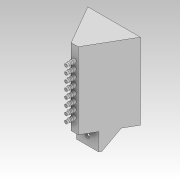
# Autodesk Inventor part: Manifold_8
Saved by Autodesk Inventor 2020 (Build 240168000, 168)
## iProperties
Created: 2020-08-02
Part Number: Manifold_8
Material: Generic
Document SubType Name: Modeling
Designer: DDeGo
Density: 1 g/cm^3
Appearance: Default
Author: DDeGo
Autodesk Inventor part; units mm, degrees
ref_plane "YZ Plane" through (0, 0, 0) normal (1, 0, 0) x (0, 1, 0)
ref_plane "XZ Plane" through (0, 0, 0) normal (0, 1, 0) x (-1, 0, 0)
ref_plane "XY Plane" through (0, 0, 0) normal (0, 0, 1) x (1, 0, 0)
sketch "Sketch1" plane through (0, 0, 0) normal (1, 0, 0) x (0, 1, 0)
  line L0 (1.75, 10) -> (1.05, 10)
  line L1 (0, 0) -> (0, 10) construction
  line L2 (0, 10) -> (1.05, 10) construction
  line L3 (1.8198, 8) -> (2.2759, 6.4097)
  line L4 (2.2759, 6.4097) -> (1.8759, 6.3957)
  line L5 (1.9282, 4.8957) -> (2.3843, 3.3053)
  line L6 (2.3843, 3.3053) -> (1.9843, 3.2914)
  line L7 (1.8759, 6.3957) -> (1.8198, 8) construction
  line L8 (1.8198, 8) -> (1.75, 10)
  line L9 (1.9282, 4.8957) -> (1.8759, 6.3957)
  line L10 (1.9843, 3.2914) -> (1.9282, 4.8957) construction
  line L11 (2.0992, 0) -> (1.9843, 3.2914)
  line L12 (1.05, 10) -> (1.05, 0)
  line L13 (1.05, 0) -> (2.0992, 0)
  line L14 (1.05, 0) -> (0, 0) construction
  dimension "d0" = 1.75
  dimension "d1" = 0.7
  dimension "d3" = 0.4
  dimension "d5" = 10
  dimension "d6" = 2
  dimension "d7" = 1.5
  dimension "d14" = 14
  dimension "d48" = 2
  constraints: 30 end point, 12 perpendicular, 2 horizontal, 2 parallel, 2 vertical
  measures "d0" distance of L1.end L0.start
  measures "d1" distance of L0.start L0.end
  measures "d3" horizontal distance of L3.end L4.end
  measures "d5" vertical distance of L11.start L0.start
  measures "d6" vertical distance of L0.end L3.start
  measures "d7" vertical distance of L4.end L5.start
  measures "d14" angle of L3 L7
  measures "d48" angle of L12 L8
revolve "Revolution1" add sketch "Sketch1" angle 360 about axis through (0, 0, 0) along (0, 0, 1)
pattern_linear "Rectangular Pattern1" count 8 spacing 8 along (0, 1, 0) of "Revolution1"
sketch "Sketch5" plane through (0, 0, 0) normal (0, 0, -1) x (-1, 0, 0)
  line L0 (4, 60) -> (-4, 60)
  line L1 (-4, 60) -> (-4, -4)
  line L2 (-4, -4) -> (4, -4)
  line L3 (4, -4) -> (4, 60)
  circle A0 centre (0, 56) radius 1.05 projected
  circle A1 centre (0, 48) radius 1.05 projected
  circle A2 centre (0, 40) radius 1.05 projected
  circle A3 centre (0, 32) radius 1.05 projected
  circle A4 centre (0, 24) radius 1.05 projected
  circle A5 centre (0, 16) radius 1.05 projected
  circle A6 centre (0, 8) radius 1.05 projected
  circle A7 centre (0, 0) radius 1.05 projected
  dimension "d50" = 4
  dimension "d51" = 4
  dimension "d55" = 4
  dimension "d56" = 4
  constraints: 8 end point, 2 parallel, 1 horizontal, 1 perpendicular
  measures "d50" distance from line of point (0, 0) L3
  measures "d51" distance from line of L1 point (0, 0)
  measures "d55" distance from line of L0 A0.centre
  measures "d56" distance from line of L2 point (0, 0)
extrude "Extrusion3" add sketch "Sketch5" along normal blind 8
ref_plane "Work Plane1" through (0, 0, -4) normal (0, 0, -1) x (-1, 0, 0)
sketch "Sketch6" plane through (-4, -4, 0) normal (0, -1, 0) x (1, 0, 0)
  line L0 (5.05, -8) -> (2.95, -8) construction
  circle A0 centre (4, -4) radius 1.75
  line L1 (9.6, -4) -> (-1.6, -4) construction
  line L2 (8, -8) -> (0, -8) projected
  line L3 (4, -8) -> (4, 0) construction
  dimension "d59" = 3.5
  constraints: 3 midpoint, 2 end point, 1 centre point, 1 coincident, 1 vertical
  measures "d59" diameter of A0
extrude "Extrusion4" cut sketch "Sketch6" against normal through all
sketch "Sketch7" plane through (0, 0, -8) normal (0, 0, -1) x (-1, 0, 0)
  circle A0 centre (0, 0) radius 1.05 projected
  line L0 (4, -4) -> (4, 60) projected
  line L1 (4, 60) -> (-4, 60) projected
  line L2 (-4, 60) -> (-4, -4) projected
  line L3 (-4, -4) -> (4, -4) projected
  circle A1 centre (0, 0) radius 1.05 projected
  circle A2 centre (0, 8) radius 1.05 projected
  circle A3 centre (0, 16) radius 1.05 projected
  circle A4 centre (0, 24) radius 1.05 projected
  circle A5 centre (0, 32) radius 1.05 projected
  circle A6 centre (0, 40) radius 1.05 projected
  circle A7 centre (0, 48) radius 1.05 projected
  circle A8 centre (0, 56) radius 1.05 projected
extrude "Extrusion5" add sketch "Sketch7" against normal up to surface contours A0 | A2 | A3 | A4 | A5 | A6 | A7 | A8 round surface about axis through (0, -4, -4) along (0, 1, 0) radius 1.75 far side no
sketch "Sketch10" plane through (-4, -4, 0) normal (0, -1, 0) x (1, 0, 0)
  line L0 (20.3187, -16.469) -> (-14.4175, -16.469)
  line L1 (-14.4175, -16.469) -> (-14.4175, -4)
  line L2 (-14.4175, -4) -> (20.3187, -4)
  line L3 (20.3187, -4) -> (20.3187, -16.469)
  circle A0 centre (4, -4) radius 1.75 projected
  point P0 (4, 0)
  constraints: 8 end point, 2 parallel, 1 horizontal, 1 perpendicular, 1 point on line
extrude "Extrusion6" cut sketch "Sketch10" against normal through all contours L0 L1 L2 A0 L3 | A0 L2 picked at (3.6188, -4.8908)
sketch "Sketch11" plane through (-4, -4, 0) normal (0, -1, 0) x (1, 0, 0)
  line L0 (4, 0) -> (4, -45) construction
  line L1 (4, -45) -> (-24.8451, -45) construction
  line L2 (-26, -45) -> (0, 0)
  line L3 (0, 0) -> (4, 0)
  arc A0 (5.75, -4) -> (2.25, -4) centre (4, -4) ccw projected
  line L4 (0, -4) -> (2.25, -4) construction
  line L5 (2.25, -4) -> (-4.3616, -9.5478)
  line L6 (-4.3616, -9.5478) -> (-24.8451, -45)
  line L7 (-24.8451, -45) -> (-26, -45)
  line L8 (34, -45) -> (8, 0)
  line L9 (8, 0) -> (4, 0)
  line L10 (5.75, -4) -> (12.3616, -9.5478)
  line L11 (12.3616, -9.5478) -> (32.8451, -45)
  line L12 (32.8451, -45) -> (34, -45)
  dimension "d90" = 45
  dimension "d92" = 30
  dimension "d93" = 40
  dimension "d94" = 1
  constraints: 24 end point, 4 symmetric about line, 2 perpendicular, 1 parallel, 1 vertical
  measures "d90" distance of L0.start L0.end
  measures "d92" distance from line of L0 L2.start
  measures "d93" angle of L4 L5
  measures "d94" distance between parallel lines of L2 L6
extrude "Extrusion7" add sketch "Sketch11" along normal blind 10
sketch "Sketch12" plane through (-4, -4, 0) normal (0, 1, 0) x (1, 0, 0)
  line L0 (0, 4) -> (2.25, 4) projected
  line L1 (-4.3616, 9.5478) -> (2.25, 4) projected
  line L2 (-24.8451, 45) -> (-4.3616, 9.5478) projected
  line L3 (-26, 45) -> (-24.8451, 45) projected
  line L4 (0, 0) -> (-26, 45) projected
  line L5 (0, 0) -> (0, 4) projected
  line L6 (5.75, 4) -> (8, 4) projected
  line L7 (8, 0) -> (8, 4) projected
  line L8 (34, 45) -> (8, 0) projected
  line L9 (32.8451, 45) -> (34, 45) projected
  line L10 (12.3616, 9.5478) -> (32.8451, 45) projected
  line L11 (5.75, 4) -> (12.3616, 9.5478) projected
  point P0 (4, 0)
extrude "Extrusion8" add sketch "Sketch12" along normal up to surface (64 mm away)
sketch "Sketch13" plane through (-4, 60, 0) normal (0, 1, 0) x (1, 0, 0)
  arc A0 (2.25, 4) -> (5.75, 4) centre (4, 4) ccw projected
  line L0 (-4.3616, 9.5478) -> (2.25, 4) projected
  line L1 (-24.8451, 45) -> (-4.3616, 9.5478) projected
  line L2 (-26, 45) -> (-24.8451, 45) projected
  line L3 (0, 0) -> (-26, 45) projected
  line L4 (0, 0) -> (8, 0) projected
  line L5 (34, 45) -> (8, 0) projected
  line L6 (32.8451, 45) -> (34, 45) projected
  line L7 (12.3616, 9.5478) -> (32.8451, 45) projected
  line L8 (5.75, 4) -> (12.3616, 9.5478) projected
  point P0 (4, 0)
extrude "Extrusion9" add sketch "Sketch13" along normal blind 10
sketch "Sketch14" plane through (-4, 70, 0) normal (0, 1, 0) x (1, 0, 0)
  line L0 (-26, 45) -> (-24.8451, 45) projected
  line L1 (8, 0) -> (34, 45) projected
  line L2 (-26, 45) -> (34, 45)
  line L3 (-26, 45) -> (0, 0) projected
  line L4 (0, 0) -> (8, 0) projected
  point P0 (4, 0)
  constraints: 2 end point, 1 horizontal
extrude "Extrusion10" add sketch "Sketch14" along normal blind 1.5
sketch "Sketch15" plane through (-4, -14, 0) normal (0, -1, 0) x (1, 0, 0)
  line L0 (8, 0) -> (34, -45) projected
  line L1 (-26, -45) -> (0, 0) projected
  line L2 (34, -45) -> (-26, -45)
  line L3 (8, 0) -> (0, 0) projected
  point P0 (4, 0)
  constraints: 2 end point, 1 horizontal
extrude "Extrusion11" add sketch "Sketch15" along normal blind 1.5
sketch "Sketch16" plane through (-4, -14, 0) normal (0, 1, 0) x (1, 0, 0)
  arc A0 (2.25, 4) -> (5.75, 4) centre (4, 4) ccw projected
  line L0 (2.25, 4) -> (5.75, 4)
  point P0 (4, 0)
  constraints: 2 end point, 1 horizontal
extrude "Extrusion12" add sketch "Sketch16" along normal blind 10
sketch "Sketch17" plane through (-4, 70, 0) normal (0, -1, 0) x (1, 0, 0)
  arc A0 (5.75, -4) -> (2.25, -4) centre (4, -4) ccw projected
  line L0 (5.75, -4) -> (2.25, -4)
  point P0 (4, 0)
  constraints: 2 end point, 1 horizontal
extrude "Extrusion13" add sketch "Sketch17" along normal blind 10
fillet "Fillet8" radius 5 8 edges at (5.0558, -14, -6.7739) (18.6033, -14, -27.2739) (-5.0558, -14, -6.7739) (-18.6033, -14, -27.2739) (5.0558, 70, -6.7739) (18.6033, 70, -27.2739) (-5.0558, 70, -6.7739) (-18.6033, 70, -27.2739)
chamfer "Chamfer1" distance 1.7 distance2 4 1 edges at (0, -4, -4) measured on face at (0, -4, -3.5)
chamfer "Chamfer2" distance 1.7 distance2 4 1 edges at (0, 60, -4) measured on face at (0, 60, -3.5)
sketch "Sketch18" plane through (-4, -15.5, 0) normal (0, -1, 0) x (1, 0, 0)
  line L0 (8, 0) -> (34, -45) construction
  line L1 (16.5, -14.7115) -> (-8.5, -14.7115)
  line L2 (-8.5, -14.7115) -> (-8.5, -17.2115)
  line L3 (-8.5, -17.2115) -> (16.5, -17.2115)
  line L4 (16.5, -17.2115) -> (16.5, -14.7115)
  line L5 (0, 0) -> (-26, -45) construction
  point P0 (4, 0)
  dimension "d113" = 25
  dimension "d114" = 2.5
  constraints: 8 end point, 2 parallel, 2 point on line, 1 horizontal, 1 perpendicular
  measures "d113" distance of L1.start L1.end
  measures "d114" distance of L1.end L2.end
extrude "Extrusion14" add sketch "Sketch18" along normal blind 20
sketch "Sketch19" plane through (-12.5, -15.5, -17.2115) normal (-1, 0, 0) x (0, 0, 1)
  line L0 (2.5, 0) -> (-27.7885, 0) construction
  line L1 (2.5, -20) -> (0, -20) projected
  line L2 (-14.0042, 0) -> (0, -20)
  line L3 (0, -20) -> (2.5, -20)
  line L4 (0, 0) -> (2.5, 0) projected
  line L5 (2.5, -20) -> (2.5, 0)
  line L6 (2.5, 0) -> (-14.0042, 0)
  point P0 (17.2115, 15.5)
  dimension "d117" = 55
  constraints: 8 end point, 2 perpendicular, 1 collinear, 1 point on line
  measures "d117" angle of L0 L2
extrude "Extrusion15" add sketch "Sketch19" along normal up to surface surface through (-4, -4, 0) normal (-0.8658651, 0, 0.5002776)
mirror "Mirror1" about plane through (0, 0, 0) normal (1, 0, 0) of "Extrusion15"
fillet "Fillet9" radius 3 3 edges at (12.5, -25.5, -17.2115) (-12.5, -25.5, -17.2115) (0, -15.5, -17.2115)
sketch "Sketch20" plane through (9.5, -35.5, -17.2115) normal (0, 0, -1) x (-1, 0, 0)
  line L0 (-3, 0) -> (22, 0) construction
  line L1 (9.5, 0) -> (9.5, 10) construction
  circle A0 centre (9.5, 10) radius 2.75
  point P0 (9.5, 35.5)
  dimension "d121" = 10
  dimension "d122" = 5.5
  constraints: 2 end point, 1 centre point, 1 coincident, 1 midpoint, 1 vertical
  measures "d121" distance of L1.start L1.end
  measures "d122" diameter of A0
extrude "Extrusion16" cut sketch "Sketch20" against normal through all
body "Solid1"
